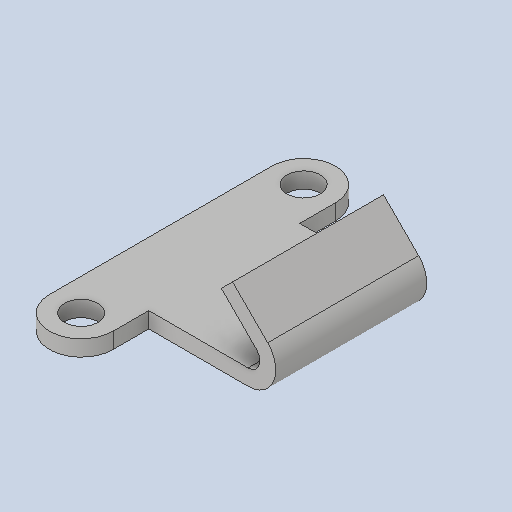
# Autodesk Inventor part: PKWS1_s
Saved by Autodesk Inventor 2024.2 (Build 282272000, 272)
## iProperties
Category: PARTsolutions
Company: MISUMI
Created: 2024-01-05
Part Number: PKWS1_s
Material: Generic
Catalog Web Link: https://jp.misumi-ec.com/vona2/detail/110300523720/?ProductCode=PKWS1
Description: PKWS_slider-Snap Locks
Vendor: MISUMI
Document SubType Name: Modeling
Designer: psAdmin
Manufacturer: MISUMI
Mass: 0.17872 g
Surface Area: 4.35849 cm^2
Volume: 0.17872 cm^3
Density: 1 g/cm^3
Appearance: PSOLRGB-175-175-175
PSOL_IDENT_0: {$CADENAS_DATA/23d-libs/misumi/metric/44_handles_hinges/pkws_slider.prj},157 {VTYP=3D},{NB=PKWS1_s},
PSOL_IDENT_1: {LINA=PKWS1},{NN=PKWS_slider},{DATE=17.04.2023 00:27:41},{GEOMDATE=04.04.2023 01:26:26},{VERSION=},{
PSOL_IDENT_2: LINEID=10},{WBVAR=},{WBNUMERIC=}  {NB=PKWS1_s},{LINA=PKWS1},{KT=DUMMY},{PN=PKWS1},{NO=1},{TL=49 (5)}
PSOL_IDENT_3: ,{MASS=11},{PPATH=assemblies_pkws\\pkws_templ.prj},{ANGLE=10.015}
NB: PKWS1_s
NN: PKWS_slider
NT: Snap Locks
NBSYN: $PN._s
LINA: PKWS1
CATALOG: Misumi
PN: PKWS1
NO: 1
TL: 49 (5)
MASS: 11
SUPPLIER: MISUMI
ARTICLENO: PKWS1_s
BOMINFO: PKWS1
CREATOR: CADENAS GmbH
Title: PKWS1
Author: Cadenas PARTsolutions
Comments: Snap Locks
Autodesk Inventor part; units mm, degrees
sketch "Sketch_1" plane through (0, 0, 0) normal (0, 0, 1) x (1, 0, 0)
  line L0 (0, 1) -> (0, 0)
  line L1 (0, 0) -> (10.25, 0)
  arc A0 (10.25, 0) -> (11.4874, 2.9874) centre (10.25, 1.75) ccw
  line L2 (11.4874, 2.9874) -> (9.2749, 5.2)
  line L3 (9.2749, 5.2) -> (8.5678, 4.4929)
  line L4 (8.5678, 4.4929) -> (10.7803, 2.2803)
  arc A1 (10.25, 1) -> (10.7803, 2.2803) centre (10.25, 1.75) ccw
  line L5 (10.25, 1) -> (0, 1)
  constraints: 12 end point, 4 point on circle, 2 centre point
extrude "Extrusion1" add sketch "Sketch_1" along normal mid plane 18
sketch "Sketch_2" plane through (0, 0, 0) normal (0, 1, 0) x (-1, 0, 0)
  line L0 (2, 11) -> (-16, 11)
  line L1 (-16, 11) -> (-16, -12)
  line L2 (-16, -12) -> (2, -12)
  line L3 (2, -12) -> (2, 11)
  line L4 (0, -7) -> (0, 7)
  arc A0 (0, 7) -> (-4, 7) centre (-2, 7) ccw
  line L5 (-4, 7) -> (-4, 4.75)
  line L6 (-4, 4.75) -> (-12, 4.75)
  line L7 (-12, 4.75) -> (-12, -4.75)
  line L8 (-12, -4.75) -> (-4, -4.75)
  line L9 (-4, -4.75) -> (-4, -7)
  arc A1 (-4, -7) -> (0, -7) centre (-2, -7) ccw
  constraints: 20 end point, 4 point on circle, 2 centre point
extrude "Extrusion2" cut sketch "Sketch_2" along normal mid plane 18
sketch "Sketch_3" plane through (0, 0, 0) normal (0, 1, 0) x (-1, 0, 0)
  circle A0 centre (-2, -7) radius 1.05
  constraints: 1 centre point
extrude "Extrusion3" cut sketch "Sketch_3" along normal mid plane 18
sketch "Sketch_4" plane through (0, 0, 0) normal (0, 1, 0) x (-1, 0, 0)
  circle A0 centre (-2, 7) radius 1.05
  constraints: 1 centre point
extrude "Extrusion4" cut sketch "Sketch_4" along normal mid plane 18
ref_plane "C_XY" through (10.1565, 1.75, 0) normal (0, 0, 1) x (1, 0, 0)
ref_plane "C_YZ" through (10.1565, 1.75, 0) normal (1, 0, 0) x (0, 1, 0)
ref_plane "C_ZX" through (10.1565, 1.75, 0) normal (0, 1, 0) x (0, 0, 1)
body "Solid1"
